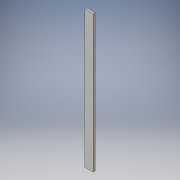
# Autodesk Inventor part: grabber articulation arms
Saved by Autodesk Inventor 2016 SP2 (Build 200236200, 236)
## iProperties
Created: 2018-02-13
Part Number: grabber articulation arms
Material: Generic
Document SubType Name: Modeling
Designer: CAD
Density: 1 g/cm^3
Appearance: Default
Author: CAD
Autodesk Inventor part; units mm, degrees
ref_plane "YZ Plane" through (0, 0, 0) normal (1, 0, 0) x (0, 1, 0)
ref_plane "XZ Plane" through (0, 0, 0) normal (0, 1, 0) x (-1, 0, 0)
ref_plane "XY Plane" through (0, 0, 0) normal (0, 0, 1) x (1, 0, 0)
sketch "Sketch1" plane through (0, 0, 0) normal (0, 1, 0) x (-1, 0, 0)
  line L0 (0, 0) -> (12.7, 0)
  line L1 (0, 0) -> (0, -3.175)
  line L2 (12.7, 0) -> (12.7, -3.175)
  line L3 (12.7, -3.175) -> (0, -3.175)
  dimension "d2" = 3.175
  dimension "d3" = 12.7
  constraints: 8 end point, 2 vertical, 1 horizontal, 1 perpendicular
  measures "d2" distance of L0.start L1.end
  measures "d3" distance of L0.start L0.end
extrude "Extrusion1" add sketch "Sketch1" along normal blind 209.55
body "Solid1"
